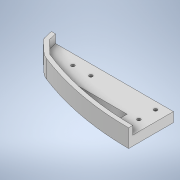
# Autodesk Inventor part: bumper_base_final _원본수정
Saved by Autodesk Inventor 2020 (Build 240168000, 168)
## iProperties
Created: 2022-06-30
Part Number: bumper_base_final _원본수정
Material: 일반
Document SubType Name: Modeling
Designer: samsung
Density: 1 g/cm^3
Appearance: 기본값
Author: samsung
Autodesk Inventor part; units mm, degrees
ref_plane "YZ Plane" through (0, 0, 0) normal (1, 0, 0) x (0, 1, 0)
ref_plane "XZ Plane" through (0, 0, 0) normal (0, 1, 0) x (-1, 0, 0)
ref_plane "XY Plane" through (0, 0, 0) normal (0, 0, 1) x (1, 0, 0)
sketch "스케치1" plane through (0, 0, 0) normal (0, 1, 0) x (-1, 0, 0)
  line L0 (-417.5, 136.0278) -> (167.5, 136.0278)
  arc A0 (126.8346, 86.699) -> (-406.6899, 73.6783) centre (-125, -531.4722) ccw
  line L1 (145.8326, 68.5278) -> (-85, 68.5278)
  line L2 (-165, 68.5278) -> (-393.8982, 68.5278)
  line L3 (-125, -531.4722) -> (-125, 1435.9267)
  circle A1 centre (-125, -531.4722) radius 1967.3989
  line L4 (-417.5444, 28.5399) -> (-406.6899, 73.6783)
  line L5 (-407.5098, 28.5399) -> (-398.3801, 66.5058)
  arc A2 (1441.9544, 38.2515) -> (-1691.7763, 38.7413) centre (-125, -531.4722) ccw
  line L6 (-371.3038, 78.1512) -> (-261.7019, 111.6599)
  line L7 (-261.7019, 111.6599) -> (11.7019, 111.6599)
  line L8 (-316.5029, 94.9056) -> (-320.1581, 106.8613)
  line L9 (-316.5029, 94.9056) -> (-397.3646, 1416.9826)
  line L10 (-316.5029, 94.9056) -> (-988.7616, 1236.1743)
  line L11 (-398.3844, 66.4971) -> (-125, -531.4722)
  line L12 (-407.5098, 28.5399) -> (-405.1717, 38.2627)
  line L13 (-405.1717, 38.2627) -> (-414.6578, 40.5439)
  line L14 (-405.1717, 38.2627) -> (-1671.8283, 684.2501)
  line L15 (-405.1717, 38.2627) -> (-2007.9181, 38.8589)
  line L16 (-405.1717, 38.2627) -> (-402.8337, 47.9856)
  line L17 (-402.8337, 47.9856) -> (-371.3038, 78.1512)
  line L18 (-387.0687, 63.0684) -> (-400.1089, 76.6983)
  line L19 (-387.0687, 63.0684) -> (-1557.9022, 816.656)
  line L20 (-387.0687, 63.0684) -> (-1051.9279, 1203.8846)
  line L21 (-125, -531.4722) -> (-261.7019, 111.6599)
  line L22 (-125, -531.4722) -> (11.7019, 111.6599)
  line L23 (-417.5444, 28.5399) -> (-407.5098, 28.5399)
  line L24 (-125, -531.4722) -> (-371.3038, 78.1512)
  line L25 (-125, -531.4722) -> (121.3038, 78.1512)
  line L26 (11.7019, 111.6599) -> (121.3038, 78.1512)
  line L27 (167.4556, 28.5399) -> (161.439, 53.6007)
  line L28 (121.3038, 78.1512) -> (152.8486, 47.9794)
  line L29 (157.5156, 28.5399) -> (167.4556, 28.5399)
  line L30 (-125, -531.4722) -> (148.2715, 66.1951)
  line L31 (-259.0118, 93.6599) -> (9.0118, 93.6599)
  line L32 (111.9521, 62.1879) -> (136.5817, 38.6304)
  line L33 (9.0118, 93.6599) -> (111.9521, 62.1879)
  line L34 (-361.9509, 62.1883) -> (-386.641, 38.5664)
  line L35 (-387.0049, 38.256) -> (-387.0101, 38.2515)
  line L36 (-388.9967, 28.5399) -> (-386.569, 38.6353)
  line L37 (-361.9509, 62.1883) -> (-259.0118, 93.6599)
  line L38 (-407.5098, 28.5399) -> (-388.9967, 28.5399)
  line L39 (136.5817, 38.6304) -> (139.0042, 28.5399)
  line L40 (157.5156, 28.5399) -> (139.0042, 28.5399)
  line L41 (-125, 111.6599) -> (-155, 111.6599)
  line L42 (-155, 111.6599) -> (-155, 93.6599)
  line L43 (-155, 93.6599) -> (-125, 93.6599)
  line L44 (-125, 93.6599) -> (-125, 111.6599)
  line L45 (152.8486, 47.9794) -> (145.0697, 46.1119)
  line L46 (145.0697, 46.1119) -> (148.5713, 31.5263)
  line L47 (148.5713, 31.5263) -> (156.3503, 33.3939)
  line L48 (137.0762, 63.0653) -> (129.8496, 69.9774)
  line L49 (129.8496, 69.9774) -> (124.32, 64.1961)
  line L50 (124.32, 64.1961) -> (138.7732, 50.372)
  line L51 (138.7732, 50.372) -> (144.3028, 56.1533)
  line L52 (66.5029, 94.9056) -> (56.9398, 97.8293)
  line L53 (56.9398, 97.8293) -> (54.6009, 90.1788)
  line L54 (54.6009, 90.1788) -> (73.727, 84.3314)
  line L55 (73.727, 84.3314) -> (76.0659, 91.9818)
  line L56 (76.0659, 91.9818) -> (66.5029, 94.9056)
  line L57 (-125, 111.6599) -> (-135, 111.6599)
  line L58 (-135, 111.6599) -> (-135, 103.6599)
  line L59 (-135, 103.6599) -> (-115, 103.6599)
  line L60 (-115, 103.6599) -> (-115, 111.6599)
  line L61 (-115, 111.6599) -> (-125, 111.6599)
  line L62 (161.439, 53.6007) -> (126.8346, 86.699)
  arc A3 (121.3038, 78.1512) -> (-398.3844, 66.4971) centre (-125, -531.4722) ccw
  line L63 (157.5156, 28.5399) -> (152.8486, 47.9794)
  line L64 (139.0042, 28.5399) -> (-125, 28.5399)
  line L65 (-85, 124.81) -> (-85, 0)
  line L66 (-125, 0) -> (-125, 61.5)
  line L67 (-125, 61.5) -> (-85, 61.5)
  line L68 (-85, 61.5) -> (-75, 61.5)
  line L69 (-75, 61.5) -> (-75, 124.1239)
  line L70 (91.215, 68.5278) -> (91.215, 89.4604)
  line L71 (-125, 28.5399) -> (-125, 78.5399)
  line L72 (-125, 78.5399) -> (91.215, 78.5399)
  line L73 (-85, 0) -> (-125, 0)
  line L74 (-75, 61.5) -> (-75, 0)
  line L75 (-75, 0) -> (-85, 0)
  line L76 (91.215, 89.4604) -> (-75, 89.4604)
  point P0 (0, 0)
  point P1 (0, 0)
  point P2 (143.8982, 61.5)
  point P3 (-393.8982, 61.5)
  point P4 (-417.5, 21.5)
  point P5 (-165, 0)
  point P6 (-85, 0)
  point P7 (-85, 12.4229)
  point P8 (167.5, 12.4229)
  point P9 (-393.8982, -388.5)
  point P10 (-165, -388.5)
  point P11 (167.5, -327)
  point P12 (-417.5, -327)
  point P13 (-85, -388.5)
  point P14 (143.8982, -388.5)
  point P15 (162, 21.5)
  point P16 (162, 12.4229)
  point P17 (167.5, 21.5)
  point P18 (-125, 0)
  point P19 (-125, 136.0278)
  point P20 (-125, 93.6599)
  point P21 (-155, 111.6599)
  point P22 (-398.3829, 66.4939)
  point P23 (128.4632, 68.5278)
  point P24 (131.3651, 68.5278)
  point P25 (-125, 103.6599)
  point P26 (143.8695, 56.5677)
  point P27 (143.1097, 54.9059)
  point P28 (-125, 126.0278)
  point P29 (-85, 28.5399)
  point P30 (-75, 68.5278)
  point P31 (-75, 78.5399)
  point P32 (-125, 136.0278)
  point P33 (-75, 28.5399)
  dimension "d13" = 667.5
  dimension "d15" = 585
  dimension "d25" = 1299.8989
  dimension "d39" = 999.8126
  dimension "d45" = 13.5
  dimension "d46" = 13.5
  dimension "d50" = 10
  dimension "d51" = 13.5
  dimension "d52" = 13.5
  dimension "d53" = 10
  dimension "d54" = 13.5
  dimension "d55" = 13.5
  dimension "d56" = 12
  dimension "d57" = 12
  dimension "d60" = 10
  dimension "d72" = 10
  dimension "d81" = 18
  dimension "d83" = 18
  dimension "d84" = 18
  dimension "d85" = 18
  dimension "d126" = 30
  dimension "d163" = 8
  dimension "d164" = 15
  dimension "d165" = 10
  dimension "d166" = 8
  dimension "d167" = 20
  dimension "d168" = 10
  dimension "d169" = 8
  dimension "d170" = 20
  dimension "d171" = 10
  dimension "d172" = 8
  dimension "d173" = 20
  dimension "d182" = 10
  dimension "d190" = 61.5
  dimension "d191" = 10
  dimension "d203" = 50
  constraints: 154 end point, 26 point on line, 23 perpendicular, 10 parallel, 8 horizontal, 6 midpoint, 6 point on circle, 2 centre point, 2 collinear, 2 vertical, 1 coincident, 1 tangent, 21 other
  measures "d13" radius of A0
  measures "d15" distance of L27.start L4.start
  measures "d39" radial gap between concentric circles of A0 A2
  measures "d45" angle of L8 L9
  measures "d46" angle of L10 L8
  measures "d50" distance of L5.start L12.end
  measures "d51" angle of L14 L13
  measures "d52" angle of L15 L13
  measures "d53" distance of L12.end L16.end
  measures "d54" angle of L18 L20
  measures "d55" angle of L18 L19
  measures "d56" angle of L3 L21
  measures "d57" angle of L22 L3
  measures "d60" angle of L24 L21
  measures "d72" angle of L25 L22
  measures "d81" distance between parallel lines of L7 L31
  measures "d83" distance between parallel lines of L28 L32
  measures "d84" distance between parallel lines of L17 L34
  measures "d85" distance between parallel lines of L12 L36
  measures "d126" distance of L42.end L43.end
  measures "d163" distance of L28.end L45.end
  measures "d164" distance of L45.end L46.end
  measures "d165" distance of L48.start L48.end
  measures "d166" distance of L48.end L49.end
  measures "d167" distance of L49.end L50.end
  measures "d168" distance of L52.start L52.end
  measures "d169" distance of L52.end L53.end
  measures "d170" distance of L53.end L54.end
  measures "d171" distance of L41.start L57.end
  measures "d172" distance of L57.end L58.end
  measures "d173" distance of L58.end L59.end
  measures "d182" distance between parallel lines of L62 L28
  measures "d190" distance of L66.start L66.end
  measures "d191" distance of L67.end L68.end
  measures "d203" distance of L64.end L71.end
extrude "돌출20" add sketch "스케치1" against normal blind 23 contours A0 L62 L1 L28 A3 L3 | A3 L65 L7 L3 | L62 L30 L28 L1 | L7 L60 L59 L3 | A3 L69 L7 L65 | L28 L30 L51 L50 L49 L1 | L1 L49 L28 | L62 L27 L29 L63 L28 L30 | L59 L60 L7 L65 L31 L3 | L7 L69 L31 L65 | L49 L50 L51 L30 L32 L25 L1 | L1 L25 L28 L49 | L28 L51 L30 | L31 L65 L72 L3 | L31 L69 L72 L65 | L25 L32 L33 L1 | L1 L70 L26 L25 | L26 L70 A3 | L28 L45 L46 L47 L63 L40 L39 L32 L30 L51 | L72 L65 L67 L3 | L70 L26 L76 | L72 L69 L1 L65 | L64 L74 L69 L1 L22 | L22 L1 L33 L32 L25 L64 | L25 L32 L30 L64 | L30 L32 L39 L64 | L1 L22 L72 L33 | L33 L72 L70 | L70 L72 L33 L76 L54 L55 L26 | L63 L47 L46 L45 | L67 L65 L64 L3 | L76 L33 L72 L22 | L22 L72 L69 L76 | L1 L69 L68 L65 | L72 L22 L1 L69 | L64 L65 L68 L74 | L76 L55 L54
extrude "돌출21" add sketch "스케치1" along normal blind 20 contours A0 L62 L1 L28 A3 L3 | L62 L30 L28 L1 | L62 L27 L29 L63 L28 L30
sketch "스케치24" plane through (125, 0, 28.5399) normal (0, 0, -1) x (-1, 0, 0)
  line L0 (0, 0) -> (50, 0) projected
  line L1 (0, 0) -> (0, -23) projected
  line L2 (50, -23) -> (0, -23)
  line L3 (50, 0) -> (50, -23) projected
  line L4 (10, -23) -> (10, -10)
  line L5 (10, -10) -> (40, -10)
  line L6 (40, -10) -> (40, -23)
  point P0 (125, 0)
  dimension "d229" = 30
  dimension "d231" = 13
  dimension "d257" = 10
  constraints: 8 end point, 1 parallel
  measures "d229" distance of L4.end L5.end
  measures "d231" distance of L4.start L4.end
  measures "d257" distance between parallel lines of L0 L5
extrude "돌출23" cut sketch "스케치24" against normal blind 32.96 contours L4 L5 L6 L2
sketch "스케치25" plane through (0, 0, 0) normal (0, 1, 0) x (1, 0, 0)
  line L0 (85, -28.5399) -> (85, -61.4999) projected
  line L1 (115, -61.4999) -> (85, -61.4999) projected
  line L2 (115, -28.5399) -> (115, -61.4999) projected
  point P0 (0, 0)
  point P1 (100, -46.4999)
  dimension "d260" = 15
  measures "d260" distance from line of point (100, -46.5) L1
hole "구멍5" at (100, 0, 46.4999) direction (0, -1, 0) diameter 4.2 end through all counterbore diameter 8 counterbore depth 5
sketch "스케치26" plane through (0, 0, 0) normal (0, 1, 0) x (1, 0, 0)
  line L0 (-157.5156, -28.5399) -> (-167.4556, -28.5399) projected
  line L1 (-152.8486, -47.9794) -> (-157.5156, -28.5399) projected
  line L2 (85, -28.5399) -> (85, -61.4999) projected
  line L3 (115, -61.4999) -> (85, -61.4999) projected
  line L4 (115, -28.5399) -> (115, -61.4999) projected
  line L5 (125, -28.5399) -> (125, -136.0278) projected
  line L6 (75, -124.1239) -> (75, -89.4604) projected
  point P0 (0, 0)
  point P1 (-91.215, -53.5399)
  point P2 (100, -86.5)
  point P3 (-48, -53.5399)
  dimension "d243" = 25
  dimension "d261" = 25.0001
  dimension "d262" = 25
  dimension "d263" = 123
  measures "d243" distance from line of L0 point (-91.215, -53.54)
  measures "d261" distance from line of point (100, -86.5) L3
  measures "d262" distance from line of L5 point (100, -86.5)
  measures "d263" distance from line of point (-48, -53.54) L6
hole "구멍6" at (-91.215, 0, 53.5399) at (100, 0, 86.5) at (-48, 0, 53.5399) direction (0, -1, 0) diameter 4.2 end through all counterbore diameter 8 counterbore depth 10
fillet "모깎기2" radius 50 1 edges at (-126.8346, -1.5, 86.699)
fillet "모깎기3" radius 10 1 edges at (-161.439, -1.5, 53.6007)
equation "\"d46\" = d45"
equation "\"d57\" = d56"
equation "\"d72\" = d60"
equation "\"d61\" = d60"
